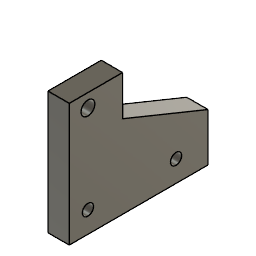
Rear Arm Pivot Bracket (Autodesk Fusion 360 design; units mm, degrees)
Autodesk Fusion 360 part; units mm, degrees
sketch "Sketch1" plane through (0, 0, 0) normal (1, 0, 0) x (0, 1, 0)
  circle A0 centre (7, 2) radius 2.1
  circle A1 centre (40, 2) radius 2.1
  line L0 (52, -6) -> (0, -6)
  line L1 (52, -6) -> (52, 12)
  circle A2 centre (7, 35) radius 2.6
  line L2 (0, 40) -> (20, 40)
  line L3 (20, 40) -> (20, 25)
  line L4 (20, 25) -> (52, 12)
  line L5 (0, 40) -> (0, -6)
  dimension "d2" = 4.2
  dimension "d4" = 4.2
  dimension "d17" = 52
  dimension "d18" = 5.2
  dimension "d19" = 20
  dimension "d20" = 46
  constraint perpendicular L0 L1
  constraint perpendicular L2 L3
  constraint perpendicular L0 L5
  measures "d2" diameter of A0
  measures "d4" diameter of A1
  measures "d17" distance of L0.start L0.end
  measures "d18" diameter of A2
  measures "d19" distance of L2.start L2.end
  measures "d20" distance of L0.end L2.start
extrude "Extrude1" add sketch "Sketch1" along normal mid plane 8
